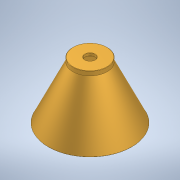
# Autodesk Inventor part: Bell
Saved by Autodesk Inventor 2021.1 (Build 251245010, 245A)
## iProperties
Created: 2025-09-17
Material: Brass, Soft Yellow
Document SubType Name: Modeling
Designer: SD
Density: 8.47 g/cm^3
Appearance: Brass - Satin
Mass: 11.6219 g
Surface Area: 28.4078 cm^2
Volume: 1.37212 cm^3
Project: Automatic Tea Steeping mechanism
Part Number: Bell
Length: 20.000 mm
BOM-Mass: 0.01162
BOM-Area: 0.003
Diameter: 30.000 mm
Author: SD
Title: Bell
Autodesk Inventor part; units mm, degrees
ref_plane "YZ Plane" through (0, 0, 0) normal (1, 0, 0) x (0, 1, 0)
ref_plane "XZ Plane" through (0, 0, 0) normal (0, 1, 0) x (-1, 0, 0)
ref_plane "XY Plane" through (0, 0, 0) normal (0, 0, 1) x (1, 0, 0)
sketch "Sketch1" plane through (0, 0, 0) normal (0, 0, 1) x (1, 0, 0)
  line L0 (0, 0) -> (0, -20) construction
  line L1 (0, 0) -> (6, 0)
  line L2 (6, 0) -> (6, -1.5)
  line L3 (6, -1.5) -> (14.6267, -20)
  line L4 (13.5233, -20) -> (4.9604, -1.6369)
  line L5 (4.9604, -1.6369) -> (4.9604, -1)
  line L6 (4.9604, -1) -> (0, -1)
  line L7 (0, 0) -> (0, -1)
  line L8 (14.6267, -20) -> (13.5233, -20)
  dimension "d1" = 6
  dimension "d2" = 1.5
  dimension "d3" = 25
  dimension "d4" = 20
  dimension "d5" = 1
  dimension "d6" = 1
  constraints: 18 end point, 3 vertical, 2 horizontal, 1 collinear, 1 point on line, 1 other
  measures "d1" distance of L0.start L1.end
  measures "d2" distance of L1.end L2.end
  measures "d3" angle of L2 L3
  measures "d4" distance from line of L3.end L1
  measures "d5" distance between parallel lines of L3 L4
  measures "d6" distance between parallel lines of L6 L1
revolve "Revolution1" add sketch "Sketch1" angle 360 about axis through (0, 0, 0) along (0, -1, 0)
chamfer "Chamfer1" distance 0.1 angle 45 3 edges at (-14.6267, -20, 0) (-13.5233, -20, 0) (-6, 0, 0)
sketch "Sketch2" plane through (0, 0, 0) normal (0, 1, 0) x (1, 0, 0)
  point P0 (0, 0)
  point P1 (0, 0)
  constraints: 1 coincident
hole "Hole1" at (0, 0, 0) direction (0, -1, 0) diameter 3.5 depth 53.6 tip angle 118
chamfer "Chamfer2" distance 0.1 angle 45 2 edges at (0, 0, -1.75) (0, -1, -1.75)
body "Solid1"
